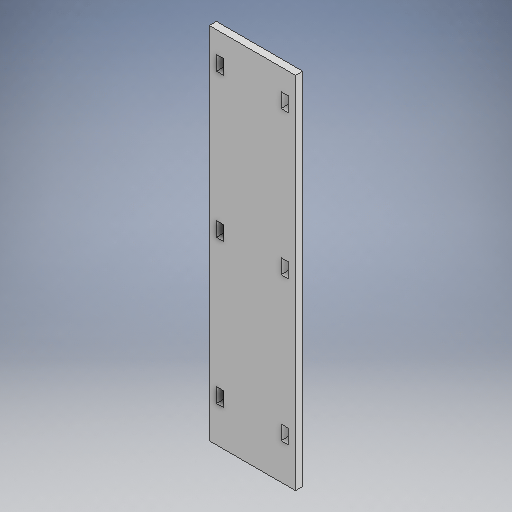
# Autodesk Inventor part: Lifting Sections right
Saved by Autodesk Inventor 2025.3 (Build 293356000, 356)
## iProperties
Created: 2026-04-06
Part Number: Lifting Sections right
Material: Generic
Document SubType Name: Modeling
Designer: user
Density: 1 g/cm^3
Appearance: Default
Author: user
Autodesk Inventor part; units mm, degrees
ref_plane "YZ Plane" through (0, 0, 0) normal (1, 0, 0) x (0, 1, 0)
ref_plane "XZ Plane" through (0, 0, 0) normal (0, 1, 0) x (-1, 0, 0)
ref_plane "XY Plane" through (0, 0, 0) normal (0, 0, 1) x (1, 0, 0)
sketch "Sketch1" plane through (0, 0, 0) normal (0, 0, 1) x (1, 0, 0)
  line L0 (-1.9934, -116.9491) -> (8.0066, -116.9491) construction
  line L1 (38.0066, 133.0509) -> (38.0066, -116.9491) construction
  line L2 (8.0066, 133.0509) -> (8.0066, -116.9491)
  line L3 (63.0066, 8.0509) -> (63.0066, -81.8491) construction
  line L4 (57.9066, 8.0509) -> (57.9066, -81.8491) construction
  line L5 (8.0066, -116.9491) -> (68.0066, -116.9491)
  line L6 (57.9066, -91.9491) -> (63.0066, -91.9491)
  line L7 (63.0066, -81.8491) -> (57.9066, -81.8491)
  line L8 (68.0066, 133.0509) -> (8.0066, 133.0509)
  line L9 (57.9066, 18.1509) -> (57.9066, 8.0509)
  line L10 (57.9066, 8.0509) -> (63.0066, 8.0509)
  line L11 (18.1066, 18.1509) -> (18.1066, 8.0509)
  line L12 (13.0066, 18.1509) -> (13.0066, 8.0509)
  line L13 (18.1066, 8.0509) -> (13.0066, 8.0509)
  line L14 (63.0066, 18.1509) -> (63.0066, 8.0509)
  line L15 (18.1066, 18.1509) -> (13.0066, 18.1509)
  line L16 (73.0066, 108.0509) -> (8.0066, 108.0509) construction
  line L17 (73.0066, 118.1509) -> (8.0066, 118.1509) construction
  line L18 (63.0066, 118.1509) -> (63.0066, 108.0509)
  line L19 (57.9066, 118.1509) -> (57.9066, 108.0509)
  line L20 (63.0066, 118.1509) -> (57.9066, 118.1509)
  line L21 (57.9066, 108.0509) -> (63.0066, 108.0509)
  line L22 (57.9066, 108.0509) -> (57.9066, 18.1509) construction
  line L23 (63.0066, 108.0509) -> (63.0066, 18.1509) construction
  line L24 (57.9066, 18.1509) -> (63.0066, 18.1509)
  line L25 (57.9066, -81.8491) -> (57.9066, -91.9491)
  line L26 (63.0066, -81.8491) -> (63.0066, -91.9491)
  line L27 (13.0066, -81.8491) -> (18.1066, -81.8491)
  line L28 (13.0066, -81.8491) -> (13.0066, -91.9491)
  line L29 (18.1066, -81.8491) -> (18.1066, -91.9491)
  line L30 (18.1066, -91.9491) -> (13.0066, -91.9491)
  line L31 (-1.9934, -91.9491) -> (68.0066, -91.9491) construction
  line L32 (8.0066, -116.9491) -> (-1.9934, -116.9491) construction
  line L33 (-1.9934, -81.8491) -> (68.0066, -81.8491) construction
  line L34 (3.0066, 108.0509) -> (68.0066, 108.0509) construction
  line L35 (3.0066, 118.1509) -> (68.0066, 118.1509) construction
  line L36 (18.1066, 108.0509) -> (13.0066, 108.0509)
  line L37 (13.0066, 118.1509) -> (13.0066, 108.0509)
  line L38 (13.0066, 118.1509) -> (18.1066, 118.1509)
  line L39 (18.1066, 118.1509) -> (18.1066, 108.0509)
  line L40 (68.0066, -116.9491) -> (68.0066, 133.0509)
  point P0 (0, 0)
  constraints: 82 end point, 18 point on line, 1 horizontal
extrude "Extrusion1" add sketch "Sketch1" along normal blind 5
body "Solid1"
